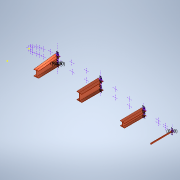
# Autodesk Inventor part: Lonjeron
Saved by Autodesk Inventor 2022 (Build 260153000, 153)
## iProperties
Created: 2022-04-09
Part Number: Lonjeron
Material: Aluminum 6061-AHC
Document SubType Name: Modeling
Designer: 40742
Density: 2.7 g/cm^3
Appearance: Metal 1400F Hot
Author: 40742
Autodesk Inventor part; units mm, degrees
ref_plane "YZ Plane" through (0, 0, 0) normal (1, 0, 0) x (0, 1, 0)
ref_plane "XZ Plane" through (0, 0, 0) normal (0, 1, 0) x (-1, 0, 0)
sketch "Sketch3" plane through (0, 0, 0) normal (0, 0, 1) x (1, 0, 0)
  point P0 (0, 0)
sketch "Sketch4" plane through (0, 0, 0) normal (0, 0, 1) x (1, 0, 0)
  line L0 (1000, -27.7533) -> (1000, 40.62) construction
  line L1 (799.98, -26.7533) -> (799.98, 74.3207) construction
  line L2 (499.94, -38.1526) -> (499.94, 116.1182) construction
  line L3 (199.94, -55.6316) -> (199.94, 130.5574) construction
  spline S0 degree 1 poles (199.94, 7.57) (204.9386, 7.6881) knots 0 0 1 1
  line L4 (199.94, 7.57) -> (194.94, 7.4474) construction
  spline S1 degree 1 poles (199.94, 7.57) (194.94, 7.4474) knots 1 1 2 2
  line L5 (194.94, 7.4474) -> (194.94, 9.4474)
  line L6 (194.94, 7.4474) -> (196.94, 7.4474) construction
  line L7 (204.9386, 7.6881) -> (204.9386, 9.6881)
  line L8 (204.9386, 7.6881) -> (206.9386, 7.6881) construction
  spline S2 degree 1 poles (199.94, 60.7036) (194.94, 60.3205) knots 0 0 1 1
  spline S3 degree 1 poles (199.94, 60.7036) (204.94, 61.0662) knots 0 0 1 1
  line L9 (194.94, 60.3205) -> (194.94, 58.3205)
  line L10 (204.94, 61.0662) -> (204.94, 59.0662)
  line L11 (200.44, 39.0539) -> (200.44, 58.7306)
  line L12 (200.44, 39.0539) -> (200.44, 9.5798)
  line L13 (200.44, 39.0539) -> (231.8058, 39.0539) construction
  line L14 (199.44, 39.0539) -> (199.44, 58.6561)
  line L15 (199.44, 39.0539) -> (199.44, 9.5557)
  line L16 (194.94, 58.3205) -> (199.44, 58.6561)
  line L17 (200.44, 58.7306) -> (204.94, 59.0662)
  line L18 (194.94, 9.4474) -> (199.44, 9.5557)
  line L19 (200.44, 9.5798) -> (204.9386, 9.6881)
  line L20 (499.94, 7.37) -> (494.94, 7.4668) construction
  spline S4 degree 1 poles (499.94, 7.37) (494.94, 7.4668) knots 1 1 2 2
  line L21 (499.94, 7.37) -> (504.94, 7.2734) construction
  spline S5 degree 1 poles (499.94, 7.37) (504.94, 7.2734) knots 1 1 2 2
  line L22 (494.94, 7.4668) -> (494.94, 9.4668)
  line L23 (504.94, 7.2734) -> (504.94, 9.2734)
  line L24 (499.94, 63.1471) -> (504.94, 63.1471) construction
  spline S6 degree 1 poles (499.94, 63.1471) (494.94, 63.3879) knots 0 0 1 1
  spline S7 degree 1 poles (499.94, 63.1471) (504.94, 62.8996) knots 0 0 1 1
  line L25 (494.94, 63.3879) -> (494.94, 61.3879)
  line L26 (504.94, 62.8996) -> (504.94, 60.8996)
  line L27 (500.44, 36.8911) -> (500.44, 61.1193)
  line L28 (500.44, 36.8911) -> (500.44, 9.3604)
  line L29 (499.44, 36.8911) -> (499.44, 61.1681)
  line L30 (499.44, 36.8911) -> (499.44, 9.3797)
  line L31 (494.94, 9.4668) -> (499.44, 9.3797)
  line L32 (500.44, 9.3604) -> (504.94, 9.2734)
  line L33 (494.94, 61.3879) -> (499.44, 61.1681)
  line L34 (500.44, 61.1193) -> (504.94, 60.8996)
  spline S8 degree 1 poles (799.98, 1.88) (794.98, 1.967) knots 0 0 1 1
  spline S9 degree 1 poles (799.98, 1.88) (804.98, 1.7938) knots 0 0 1 1
  line L35 (794.98, 1.967) -> (794.98, 3.967)
  line L36 (804.98, 1.7938) -> (804.98, 3.7938)
  spline S10 degree 1 poles (799.98, 33.5425) (794.98, 34.2602) knots 0 0 1 1
  spline S11 degree 1 poles (799.98, 33.5425) (804.98, 32.8164) knots 0 0 1 1
  line L37 (794.98, 34.2602) -> (794.98, 32.2602)
  line L38 (804.98, 32.8164) -> (804.98, 30.8164)
  line L39 (800.48, 21.2767) -> (800.48, 31.4661)
  line L40 (800.48, 21.2767) -> (800.48, 3.8717)
  line L41 (799.48, 21.2767) -> (799.48, 31.6105)
  line L42 (799.48, 21.2767) -> (799.48, 3.8891)
  line L43 (794.98, 32.2602) -> (799.48, 31.6105)
  line L44 (800.48, 31.4661) -> (804.98, 30.8164)
  line L45 (794.98, 3.967) -> (799.48, 3.8891)
  line L46 (800.48, 3.8717) -> (804.98, 3.7938)
  line L47 (995, 2.6819) -> (995, -1.7332)
  line L48 (995, -1.7332) -> (997, -1.7332)
  line L49 (995, -1.7332) -> (997, -1.7332) construction
  line L50 (997, -1.7332) -> (997, 2.3108)
  spline S12 degree 1 poles (995, 2.6819) (997, 2.3108) knots 0 0 1 1
  point P0 (0, 0)
  point P1 (1000, 1.75)
  point P2 (949.91, 10.33)
  point P3 (899.85, 18.11)
  point P4 (799.72, 33.58)
  point P5 (699.61, 46.34)
  point P6 (599.53, 56.61)
  point P7 (499.47, 63.17)
  point P8 (399.44, 66.64)
  point P9 (299.45, 65.8)
  point P10 (199.49, 60.67)
  point P11 (149.54, 55.65)
  point P12 (99.6, 47.73)
  point P13 (74.65, 41.62)
  point P14 (49.72, 33.92)
  point P15 (24.81, 23.11)
  point P16 (12.36, 16.6)
  point P17 (0, 0)
  point P18 (12.58, -9.99)
  point P19 (25.08, -9.39)
  point P20 (50.04, -4.68)
  point P21 (75.01, -1.47)
  point P22 (99.99, 1.33)
  point P23 (149.95, 5.55)
  point P24 (299.92, 9.6)
  point P25 (399.92, 9.24)
  point P26 (599.95, 5.51)
  point P27 (699.97, 3.74)
  point P28 (900, 0.11)
  point P29 (950.01, -1.07)
  point P30 (1000, -1.75)
  dimension "d35" = 2
  dimension "d36" = 90
  dimension "d37" = 2
  dimension "d38" = 90
  dimension "d43" = 2
  dimension "d44" = 2
  dimension "d51" = 2
  dimension "d52" = 2
  dimension "d56" = 2
  dimension "d57" = 2
  dimension "d65" = 2
  dimension "d66" = 2
  dimension "d69" = 2
  dimension "d70" = 2
  dimension "d76" = 2
  dimension "d77" = 0
  constraints: 96 end point, 20 vertical, 6 horizontal, 5 coincident, 3 equal length, 3 parallel, 3 point on line, 1 perpendicular, 30 other
  measures "d35" distance of L4.end L5.end
  measures "d36" angle of L6 L5
  measures "d37" distance of L7.start L7.end
  measures "d38" angle of L8 L7
  measures "d43" distance of L9.start L9.end
  measures "d44" distance of L10.start L10.end
  measures "d51" distance of L20.end L22.end
  measures "d52" distance of L21.end L23.end
  measures "d56" distance of L25.start L25.end
  measures "d57" distance of L26.start L26.end
  measures "d65" distance of L35.start L35.end
  measures "d66" distance of L36.start L36.end
  measures "d69" distance of L37.start L37.end
  measures "d70" distance of L38.start L38.end
  measures "d76" distance of L47.end L48.end
  measures "d77" distance between parallel lines of L48 L49
sketch "Sketch5" plane through (0, 0, 0) normal (0, 0, 1) x (1, 0, 0)
  point P0 (0, 0)
sketch "Sketch6" plane through (0, 0, 0) normal (0, 0, 1) x (1, 0, 0)
  point P0 (0, 0)
ref_plane "Work Plane2" through (0, 0, 150) normal (0, 0, 1) x (1, 0, 0)
sketch "Sketch9" plane through (0, 0, 150) normal (0, 0, 1) x (1, 0, 0)
  point P0 (0, 0)
sketch "Sketch10" plane through (0, 0, 150) normal (0, 0, 1) x (1, 0, 0)
  line L0 (1000, -15.7401) -> (1000, 30.353) construction
  spline S0 degree 4 poles (1000, 1.4) (958.0806, 9.2692) (944.7397, 9.7911) (832.8033, 29.6403) (729.9887, 41.5892) (638.7953, 51.8217) (550.8542, 57.0203) (458.4327, 60.5557) (382.8343, 60.3203) (282.3638, 55.2323) (247.4759, 51.7518) (192.2324, 44.5633) (169.7365, 37.5042) (147.9718, 33.0302) (120.8385, 19.2072) (114.8492, 18.6016) (90.37, -0.7829) (114.6478, -12.4462) (121.6476, -7.8197) (148.9968, -3.6688) (170.9929, -1.0634) (199.4125, 2.1652) (250.8296, 6.9694) (385.6616, 9.037) (451.9997, 8.4981) (550.9389, 6.3783) (638.6063, 4.7866) (730.2764, 3.2267) (832.6338, 1.2406) (944.8733, -0.7521) (958.1113, -0.6568) (1000, -3.8763) knots 0 0 0 0 0 0.083942 0.123015 0.165125 0.207171 0.249169 0.29114 0.330039 0.365904 0.396598 0.422157 0.44575 0.465817 0.48534 0.503709 0.520324 0.538292 0.556752 0.576267 0.599497 0.630287 0.666301 0.707547 0.751855 0.793808 0.835762 0.877715 0.916598 1 1 1 1 1 construction
  spline S1 degree 1 poles (549.946, 6.458) (554.446, 6.3698) knots 0 0 1 1 construction
  line L1 (554.446, 56.4347) -> (556.246, 56.4347) construction
  line L2 (1000, -3.8763) -> (1004.5, -3.8763) construction
  spline S2 degree 1 poles (997.3, -3.6709) (995.5, -3.534) knots 0 0 1 1
  line L3 (1000, 1.4) -> (1004.5, 1.4) construction
  spline S3 degree 1 poles (997.3, 1.9032) (995.5, 2.2387) knots 0 0 1 1
  line L4 (995.5, -3.534) -> (997.3, -3.534) construction
  line L5 (997.3, -3.534) -> (997.3, -3.6709)
  line L6 (997.3, -3.6709) -> (997.3, 1.9047)
  line L7 (995.5, 2.2387) -> (995.5, -3.534)
  line L8 (997.759, -3.7058) -> (996.841, -3.636) construction
  arc A0 (996.9328, -3.643) -> (997.6672, -3.6988) centre (1755.7279, 9967.527) ccw construction
  line L9 (997.759, 1.8177) -> (996.841, 1.9887) construction
  arc A1 (996.9328, 1.9716) -> (997.6672, 1.8348) centre (2829.4709, 9832.628) ccw construction
  spline S4 degree 1 poles (800.48, 1.8802) (795.98, 1.9644) knots 0 0 1 1
  spline S5 degree 1 poles (800.48, 1.8802) (804.98, 1.796) knots 0 0 1 1
  line L10 (804.98, 1.796) -> (804.98, 3.596)
  line L11 (795.98, 1.9644) -> (795.98, 3.7644)
  line L12 (800.48, 1.8802) -> (800.48, 42.782) construction
  line L13 (800.48, 32.7554) -> (804.98, 32.7554) construction
  spline S6 degree 1 poles (800.48, 32.7554) (804.98, 32.1362) knots 0 0 1 1
  spline S7 degree 1 poles (800.48, 32.7554) (795.98, 33.3662) knots 0 0 1 1
  line L14 (795.98, 33.3662) -> (795.98, 31.5662)
  line L15 (804.98, 32.1362) -> (804.98, 30.3362)
  line L16 (800.93, 20.0905) -> (800.93, 30.8897)
  line L17 (800.93, 20.0905) -> (800.93, 3.6718)
  line L18 (800.48, 20.0905) -> (800.93, 20.0905) construction
  line L19 (800.03, 20.0905) -> (800.03, 31.0127)
  line L20 (800.03, 20.0905) -> (800.03, 3.6886)
  line L21 (795.98, 31.5662) -> (800.03, 31.0127)
  line L22 (800.93, 30.8897) -> (804.98, 30.3362)
  line L23 (795.98, 3.7644) -> (800.03, 3.6886)
  line L24 (800.93, 3.6718) -> (804.98, 3.596)
  line L25 (1000, -8.626) -> (1495.05, -8.626) construction
  line L26 (500.45, 7.4293) -> (504.95, 7.3436) construction
  spline S8 degree 1 poles (500.45, 7.4293) (504.95, 7.3436) knots 1 1 2 2
  line L27 (500.45, 7.4293) -> (495.95, 7.5149) construction
  spline S9 degree 1 poles (500.45, 7.4293) (495.95, 7.5149) knots 1 1 2 2
  line L28 (504.95, 7.3436) -> (504.95, 9.1436)
  line L29 (504.95, 7.3436) -> (506.75, 7.3436) construction
  line L30 (495.95, 7.5149) -> (495.95, 9.3149)
  line L31 (495.95, 7.5149) -> (497.75, 7.5149) construction
  line L32 (500.45, 7.4293) -> (500.45, 71.956) construction
  spline S10 degree 1 poles (500.45, 58.7181) (504.95, 58.5609) knots 0 0 1 1
  spline S11 degree 1 poles (500.45, 58.7181) (495.95, 58.8687) knots 0 0 1 1
  line L33 (504.95, 58.5609) -> (504.95, 56.7609)
  line L34 (495.95, 58.8687) -> (495.95, 57.0687)
  line L35 (500.45, 42.5087) -> (500.9, 42.5087) construction
  line L36 (500.9, 42.5087) -> (500.9, 56.8994)
  line L37 (500.9, 42.5087) -> (500.9, 9.2207)
  line L38 (500.45, 31.5662) -> (500.9, 31.5662) construction
  line L39 (500, 31.5662) -> (500, 9.2378)
  line L40 (500, 31.5662) -> (500, 56.9302)
  line L41 (495.95, 57.0687) -> (500, 56.9302)
  line L42 (500.9, 56.8994) -> (504.95, 56.7609)
  line L43 (495.95, 9.3149) -> (500, 9.2378)
  line L44 (500.9, 9.2207) -> (504.95, 9.1436)
  line L45 (1000, -11.9137) -> (1795.061, -11.9137) construction
  spline S12 degree 1 poles (200.439, 2.0881) (204.939, 2.517) knots 0 0 1 1
  spline S13 degree 1 poles (200.439, 2.0881) (195.939, 1.64) knots 0 0 1 1
  line L46 (204.939, 2.517) -> (204.939, 4.317)
  line L47 (195.939, 1.64) -> (195.939, 3.44)
  spline S14 degree 1 poles (200.439, 44.8907) (195.939, 44.0576) knots 0 0 1 1
  spline S15 degree 1 poles (200.439, 44.8907) (204.939, 45.6685) knots 0 0 1 1
  line L48 (195.939, 44.0576) -> (195.939, 42.2576)
  line L49 (195.939, 44.0576) -> (197.739, 44.0576) construction
  line L50 (204.939, 45.6685) -> (204.939, 43.8685)
  line L51 (204.939, 45.6685) -> (206.739, 45.6685) construction
  line L52 (200.439, 44.8907) -> (200.439, 2.0881) construction
  line L53 (200.889, 14.9404) -> (200.889, 3.9224)
  line L54 (200.889, 14.9404) -> (200.889, 43.1436)
  line L55 (200.439, 14.9404) -> (200.889, 14.9404) construction
  line L56 (199.989, 14.9404) -> (199.989, 42.9825)
  line L57 (199.989, 14.9404) -> (199.989, 3.8347)
  line L58 (195.939, 3.44) -> (199.989, 3.8347)
  line L59 (200.889, 3.9224) -> (204.939, 4.317)
  line L60 (204.939, 43.8685) -> (200.889, 43.1436)
  line L61 (199.989, 42.9825) -> (195.939, 42.2576)
  point P0 (0, 0)
  point P1 (0, 0)
  point P2 (954.919, 9.122)
  point P3 (909.865, 16.124)
  point P4 (819.748, 30.047)
  point P5 (729.649, 41.531)
  point P6 (639.577, 50.774)
  point P7 (459.496, 59.801)
  point P8 (369.505, 59.045)
  point P9 (279.541, 54.428)
  point P10 (234.586, 49.91)
  point P11 (189.64, 42.782)
  point P12 (167.185, 37.283)
  point P13 (144.748, 30.353)
  point P14 (122.329, 20.624)
  point P15 (111.124, 14.765)
  point P16 (100, -0.175)
  point P17 (111.322, -9.166)
  point P18 (122.572, -8.626)
  point P19 (145.036, -4.387)
  point P20 (167.509, -1.498)
  point P21 (189.991, 1.022)
  point P22 (234.955, 4.82)
  point P23 (279.946, 6.638)
  point P24 (369.928, 8.465)
  point P25 (459.928, 8.141)
  point P26 (639.955, 4.784)
  point P27 (729.973, 3.191)
  point P28 (819.982, 1.517)
  point P29 (910, -0.076)
  point P30 (955.009, -1.138)
  point P31 (275.446, 6.5276)
  point P32 (284.446, 6.7443)
  point P33 (275.446, 54.1135)
  point P34 (284.446, 54.7846)
  point P35 (545.446, 6.5465)
  point P36 (545.446, 56.8741)
  point P37 (815.482, 1.6004)
  point P38 (824.482, 1.4338)
  point P39 (815.482, 30.6592)
  point P40 (824.482, 29.3598)
  point P41 (504.95, 7.3427)
  dimension "d150" = 1.8
  dimension "d151" = 1.8
  dimension "d156" = 1.8
  dimension "d157" = 1.8
  dimension "d167" = 1.8
  dimension "d168" = 90
  dimension "d169" = 1.8
  dimension "d170" = 90
  dimension "d175" = 1.8
  dimension "d176" = 1.8
  dimension "d187" = 1.8
  dimension "d188" = 1.8
  dimension "d193" = 1.8
  dimension "d194" = 90
  dimension "d195" = 1.8
  dimension "d196" = 90
  constraints: 120 end point, 25 vertical, 15 horizontal, 10 point on line, 4 midpoint, 4 perpendicular, 2 centre point, 2 point on circle, 1 collinear, 1 parallel, 1 vertical alignment, 97 other
  measures "d150" distance of L10.start L10.end
  measures "d151" distance of L11.start L11.end
  measures "d156" distance of L14.start L14.end
  measures "d157" distance of L15.start L15.end
  measures "d167" distance of L26.end L28.end
  measures "d168" angle of L29 L28
  measures "d169" distance of L27.end L30.end
  measures "d170" angle of L31 L30
  measures "d175" distance of L33.start L33.end
  measures "d176" distance of L34.start L34.end
  measures "d187" distance of L46.start L46.end
  measures "d188" distance of L47.start L47.end
  measures "d193" distance of L48.start L48.end
  measures "d194" angle of L48 L49
  measures "d195" distance of L50.start L50.end
  measures "d196" angle of L50 L51
sketch "Sketch14" plane through (0, 0, 150) normal (0, 0, 1) x (1, 0, 0)
  line L0 (200.439, 2.0881) -> (204.939, 2.517) projected
  line L1 (200.439, 2.0881) -> (195.939, 1.64) projected
  line L2 (195.939, 1.64) -> (195.939, 3.44) projected
  line L3 (195.939, 3.44) -> (199.989, 3.8347) projected
  line L4 (200.889, 3.9224) -> (204.939, 4.317) projected
  line L5 (204.939, 2.517) -> (204.939, 4.317) projected
  line L6 (200.889, 14.9404) -> (200.889, 3.9224) projected
  line L7 (199.989, 14.9404) -> (199.989, 3.8347) projected
  line L8 (200.889, 14.9404) -> (200.889, 43.1436) projected
  line L9 (199.989, 14.9404) -> (199.989, 42.9825) projected
  line L10 (204.939, 43.8685) -> (200.889, 43.1436) projected
  line L11 (204.939, 45.6685) -> (204.939, 43.8685) projected
  line L12 (200.439, 44.8907) -> (204.939, 45.6685) projected
  line L13 (200.439, 44.8907) -> (195.939, 44.0576) projected
  line L14 (195.939, 44.0576) -> (195.939, 42.2576) projected
  line L15 (199.989, 42.9825) -> (195.939, 42.2576) projected
  point P0 (0, 0)
sketch "Sketch15" plane through (0, 0, 150) normal (0, 0, 1) x (1, 0, 0)
  line L0 (504.95, 7.3436) -> (504.95, 9.1436) projected
  line L1 (500.45, 7.4293) -> (504.95, 7.3436) projected
  line L2 (500.9, 9.2207) -> (504.95, 9.1436) projected
  line L3 (495.95, 9.3149) -> (500, 9.2378) projected
  line L4 (495.95, 7.5149) -> (495.95, 9.3149) projected
  line L5 (500.45, 7.4293) -> (495.95, 7.5149) projected
  line L6 (500.9, 42.5087) -> (500.9, 9.2207) projected
  line L7 (500, 31.5662) -> (500, 9.2378) projected
  line L8 (500, 31.5662) -> (500, 56.9302) projected
  line L9 (500.9, 42.5087) -> (500.9, 56.8994) projected
  line L10 (504.95, 58.5609) -> (504.95, 56.7609) projected
  line L11 (500.45, 58.7181) -> (504.95, 58.5609) projected
  line L12 (500.45, 58.7181) -> (495.95, 58.8687) projected
  line L13 (495.95, 58.8687) -> (495.95, 57.0687) projected
  line L14 (495.95, 57.0687) -> (500, 56.9302) projected
  line L15 (500.9, 56.8994) -> (504.95, 56.7609) projected
  point P0 (0, 0)
sketch "Sketch16" plane through (0, 0, 150) normal (0, 0, 1) x (1, 0, 0)
  line L0 (800.93, 3.6718) -> (804.98, 3.596) projected
  line L1 (804.98, 1.796) -> (804.98, 3.596) projected
  line L2 (800.48, 1.8802) -> (804.98, 1.796) projected
  line L3 (800.48, 1.8802) -> (795.98, 1.9644) projected
  line L4 (795.98, 1.9644) -> (795.98, 3.7644) projected
  line L5 (795.98, 3.7644) -> (800.03, 3.6886) projected
  line L6 (800.03, 20.0905) -> (800.03, 3.6886) projected
  line L7 (800.93, 20.0905) -> (800.93, 3.6718) projected
  line L8 (800.93, 20.0905) -> (800.93, 30.8897) projected
  line L9 (800.03, 20.0905) -> (800.03, 31.0127) projected
  line L10 (795.98, 31.5662) -> (800.03, 31.0127) projected
  line L11 (800.93, 30.8897) -> (804.98, 30.3362) projected
  line L12 (804.98, 32.1362) -> (804.98, 30.3362) projected
  line L13 (800.48, 32.7554) -> (804.98, 32.1362) projected
  line L14 (800.48, 32.7554) -> (795.98, 33.3662) projected
  line L15 (795.98, 33.3662) -> (795.98, 31.5662) projected
  point P0 (0, 0)
sketch "Sketch17" plane through (0, 0, 150) normal (0, 0, 1) x (1, 0, 0)
  line L0 (997.3, -3.6709) -> (997.3, 1.9047) projected
  line L1 (997.3, -3.6709) -> (995.5, -3.534) projected
  line L2 (995.5, 2.2387) -> (995.5, -3.534) projected
  line L3 (997.3, 1.9032) -> (995.5, 2.2387) projected
  point P0 (0, 0)
sketch "Sketch18" plane through (0, 0, 0) normal (0, 0, 1) x (1, 0, 0)
  line L0 (204.9386, 7.6881) -> (204.9386, 9.6881) projected
  line L1 (199.94, 7.57) -> (204.9386, 7.6881) projected
  line L2 (199.94, 7.57) -> (194.94, 7.4474) projected
  line L3 (194.94, 7.4474) -> (194.94, 9.4474) projected
  line L4 (194.94, 9.4474) -> (199.44, 9.5557) projected
  line L5 (200.44, 9.5798) -> (204.9386, 9.6881) projected
  line L6 (200.44, 39.0539) -> (200.44, 9.5798) projected
  line L7 (199.44, 39.0539) -> (199.44, 9.5557) projected
  line L8 (200.44, 39.0539) -> (200.44, 58.7306) projected
  line L9 (199.44, 39.0539) -> (199.44, 58.6561) projected
  line L10 (194.94, 58.3205) -> (199.44, 58.6561) projected
  line L11 (194.94, 60.3205) -> (194.94, 58.3205) projected
  line L12 (199.94, 60.7036) -> (194.94, 60.3205) projected
  line L13 (199.94, 60.7036) -> (204.94, 61.0662) projected
  line L14 (204.94, 61.0662) -> (204.94, 59.0662) projected
  line L15 (200.44, 58.7306) -> (204.94, 59.0662) projected
  point P0 (0, 0)
sketch "Sketch19" plane through (0, 0, 0) normal (0, 0, 1) x (1, 0, 0)
  line L0 (504.94, 7.2734) -> (504.94, 9.2734) projected
  line L1 (499.94, 7.37) -> (504.94, 7.2734) projected
  line L2 (499.94, 7.37) -> (494.94, 7.4668) projected
  line L3 (494.94, 7.4668) -> (494.94, 9.4668) projected
  line L4 (494.94, 9.4668) -> (499.44, 9.3797) projected
  line L5 (500.44, 9.3604) -> (504.94, 9.2734) projected
  line L6 (500.44, 36.8911) -> (500.44, 9.3604) projected
  line L7 (499.44, 36.8911) -> (499.44, 9.3797) projected
  line L8 (500.44, 36.8911) -> (500.44, 61.1193) projected
  line L9 (499.44, 36.8911) -> (499.44, 61.1681) projected
  line L10 (500.44, 61.1193) -> (504.94, 60.8996) projected
  line L11 (504.94, 62.8996) -> (504.94, 60.8996) projected
  line L12 (499.94, 63.1471) -> (504.94, 62.8996) projected
  line L13 (499.94, 63.1471) -> (494.94, 63.3879) projected
  line L14 (494.94, 63.3879) -> (494.94, 61.3879) projected
  line L15 (494.94, 61.3879) -> (499.44, 61.1681) projected
  point P0 (0, 0)
sketch "Sketch20" plane through (0, 0, 0) normal (0, 0, 1) x (1, 0, 0)
  line L0 (804.98, 1.7938) -> (804.98, 3.7938) projected
  line L1 (799.98, 1.88) -> (804.98, 1.7938) projected
  line L2 (800.48, 3.8717) -> (804.98, 3.7938) projected
  line L3 (794.98, 3.967) -> (799.48, 3.8891) projected
  line L4 (794.98, 1.967) -> (794.98, 3.967) projected
  line L5 (799.98, 1.88) -> (794.98, 1.967) projected
  line L6 (799.48, 21.2767) -> (799.48, 3.8891) projected
  line L7 (800.48, 21.2767) -> (800.48, 3.8717) projected
  line L8 (800.48, 21.2767) -> (800.48, 31.4661) projected
  line L9 (799.48, 21.2767) -> (799.48, 31.6105) projected
  line L10 (794.98, 32.2602) -> (799.48, 31.6105) projected
  line L11 (794.98, 34.2602) -> (794.98, 32.2602) projected
  line L12 (799.98, 33.5425) -> (794.98, 34.2602) projected
  line L13 (799.98, 33.5425) -> (804.98, 32.8164) projected
  line L14 (804.98, 32.8164) -> (804.98, 30.8164) projected
  line L15 (800.48, 31.4661) -> (804.98, 30.8164) projected
  point P0 (0, 0)
sketch "Sketch21" plane through (0, 0, 0) normal (0, 0, 1) x (1, 0, 0)
  line L0 (997, -1.7332) -> (997, 2.3108) projected
  line L1 (995, -1.7332) -> (997, -1.7332) projected
  line L2 (995, 2.6819) -> (995, -1.7332) projected
  line L3 (995, 2.6819) -> (997, 2.3108) projected
  point P0 (0, 0)
loft "Loft2" add profiles "Sketch18", "Sketch14"
loft "Loft3" add profiles "Sketch19", "Sketch15"
loft "Loft4" add profiles "Sketch20", "Sketch16"
loft "Loft5" add profiles "Sketch21", "Sketch17"
thicken "Thicken2" operation add thickness 12.5 both sides no extend neighbours yes toward (1, 0, -0.0000026) faces at (204.9387, 6.6089, 50)
thicken "Thicken3" operation add thickness 12.5 both sides no extend neighbours yes toward (1, 0, 0.0000067) faces at (204.9397, 54.6447, 50)
thicken "Thicken4" operation add thickness 12.5 both sides no extend neighbours yes toward (-0.9999778, 0, 0.0066599) faces at (195.273, 53.6106, 50)
thicken "Thicken5" operation add thickness 12.5 both sides no extend neighbours yes toward (-0.9999778, 0, 0.0066599) faces at (195.273, 6.7783, 50)
thicken "Thicken6" operation add thickness 12.5 both sides no extend neighbours yes toward (1, 0, -0.0000667) faces at (504.9433, 60.8089, 50)
thicken "Thicken7" operation add thickness 12.5 both sides no extend neighbours yes toward (1, 0, -0.0000668) faces at (504.9433, 8.5857, 50)
thicken "Thicken8" operation add thickness 12.5 both sides no extend neighbours yes toward (-0.9999773, 0, 0.0067332) faces at (495.2767, 60.5926, 50)
thicken "Thicken9" operation add thickness 12.5 both sides no extend neighbours yes toward (-0.9999773, 0, 0.0067332) faces at (495.2767, 8.1273, 50)
thicken "Thicken10" operation add thickness 10 both sides no extend neighbours yes toward (1, 0, 0) faces at (804.98, 31.3008, 50)
thicken "Thicken12" operation add thickness 10 both sides no extend neighbours yes toward (-0.9999778, 0, 0.0066665) faces at (795.3133, 2.6106, 50)
thicken "Thicken13" operation add thickness 10 both sides no extend neighbours yes toward (-0.9999778, 0, 0.0066665) faces at (795.3133, 33.3178, 50)
thicken "Thicken14" operation add thickness 10 both sides no extend neighbours yes toward (1, 0, 0) faces at (804.98, 3.0834, 50)
sketch "Sketch22" plane through (0, 0, 150) normal (0, 0, 1) x (1, 0, 0)
  line L0 (997.3, -3.6709) -> (1000, -3.8763) construction
  spline S0 degree 1 poles (997.3, -3.6709) (1000, -3.8763) knots 1 1 2 2
  line L1 (997.3, 1.9032) -> (1000, 1.4) construction
  spline S1 degree 1 poles (997.3, 1.9032) (1000, 1.4) knots 1 1 2 2
  line L2 (997.3, 1.9032) -> (997.3, -3.6709)
  line L3 (1000, 1.4) -> (1000, -3.8763)
  point P0 (0, 0)
  constraints: 4 end point, 1 parallel, 1 vertical, 6 other
sketch "Sketch23" plane through (0, 0, 0) normal (0, 0, 1) x (1, 0, 0)
  point P0 (0, 0)
  point P1 (1000, -1.75)
  point P2 (997, -1.7332)
  point P3 (997, 2.3108)
sketch "Sketch24" plane through (0, 0, 0) normal (0, 0, 1) x (1, 0, 0)
  spline S0 degree 1 poles (1000, -1.75) (997, -1.7332) knots 0 0 1 1
  spline S1 degree 1 poles (1000, 1.75) (997, 2.3108) knots 0 0 1 1
  line L0 (1000, 1.75) -> (1000, -1.75)
  line L1 (997, 2.3108) -> (997, -1.7332)
  point P0 (0, 0)
  constraints: 4 end point, 2 vertical, 4 other
loft "Loft6" add profiles "Sketch24", "Sketch22"
body "Solid4"
